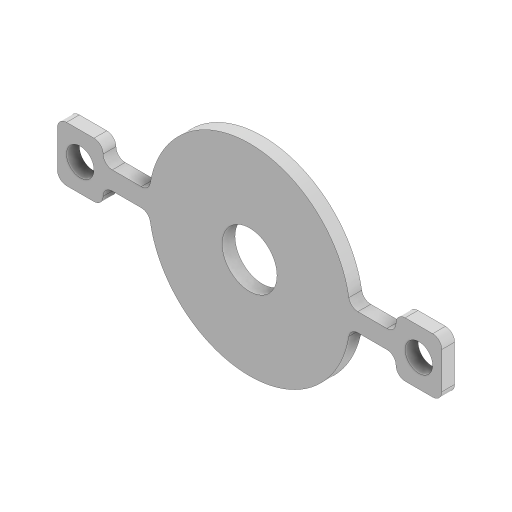
# Autodesk Inventor part: TAPA QUE DESPLAZA CON TORNILLOS
Saved by Autodesk Inventor 2024 (Build 280153000, 153)
## iProperties
Created: 2024-05-26
Part Number: TAPA QUE DESPLAZA CON TORNILLOS
Material: Generic
Document SubType Name: Modeling
Designer: Jhuliams
Density: 1 g/cm^3
Appearance: Default
Author: Jhuliams
Autodesk Inventor part; units mm, degrees
ref_plane "YZ Plane" through (0, 0, 0) normal (1, 0, 0) x (0, 1, 0)
ref_plane "XZ Plane" through (0, 0, 0) normal (0, 1, 0) x (-1, 0, 0)
ref_plane "XY Plane" through (0, 0, 0) normal (0, 0, 1) x (1, 0, 0)
sketch "Sketch1" plane through (0, 0, 0) normal (0, 0, 1) x (1, 0, 0)
  circle A0 centre (0, 0) radius 55
  line L0 (0, 0) -> (0, 20) construction
  line L1 (5, 15) -> (105, 15)
  line L2 (105, 15) -> (105, -15)
  line L3 (105, -15) -> (5, -15)
  line L4 (5, -15) -> (5, 15)
  line L5 (5, 15) -> (105, -15) construction
  line L6 (105, 15) -> (5, -15) construction
  line L7 (30, 5) -> (80, 5)
  line L8 (80, 5) -> (80, -5)
  line L9 (80, -5) -> (30, -5)
  line L10 (30, -5) -> (30, 5)
  line L11 (30, 5) -> (80, -5) construction
  line L12 (80, 5) -> (30, -5) construction
  line L13 (80, 5) -> (80, 15)
  line L14 (80, -5) -> (80, -15)
  line L15 (-5, 15) -> (-105, 15)
  line L16 (-105, 15) -> (-105, -15)
  line L17 (-105, -15) -> (-5, -15)
  line L18 (-5, -15) -> (-5, 15)
  line L19 (-5, 15) -> (-105, -15) construction
  line L20 (-105, 15) -> (-5, -15) construction
  line L21 (-30, 5) -> (-80, 5)
  line L22 (-80, 5) -> (-80, -5)
  line L23 (-80, -5) -> (-30, -5)
  line L24 (-30, -5) -> (-30, 5)
  line L25 (-30, 5) -> (-80, -5) construction
  line L26 (-80, 5) -> (-30, -5) construction
  line L27 (-80, 5) -> (-80, 15)
  line L28 (-80, -5) -> (-80, -15)
  point P0 (55, 0)
  point P1 (55, 0)
  point P2 (-55, 0)
  point P3 (-55, 0)
  point P4 (54.7723, 5)
  point P5 (54.7723, -5)
  point P6 (-54.7723, -5)
  point P7 (-54.7723, 5)
  dimension "d0" = 110
  dimension "d3" = 20
  dimension "d17" = 100
  dimension "d18" = 30
  dimension "d19" = 50
  dimension "d20" = 10
  constraints: 58 end point, 12 symmetric about line, 5 midpoint, 4 parallel, 4 perpendicular, 4 point on line, 2 horizontal, 1 coincident, 1 vertical, 3 other
  measures "d3" distance of L0.start L0.end
  measures "d17" distance of L2.end L3.end
  measures "d18" distance of L1.end L2.end
  measures "d19" distance of L8.end L9.end
  measures "d20" distance of L7.end L8.end
extrude "Extrusion1" add sketch "Sketch1" along normal blind 7 contours A0 L9 L10 L7 | A0 L7 L8 L9 | L7 L10 L9 A0 L3 L4 L1 | L1 L4 L3 A0 L17 L18 L15 | L13 L1 L2 L3 L14 L8 | L15 L18 L17 A0 L23 L24 L21 | L21 L24 L23 A0 | A0 L23 L22 L21 | L27 L22 L28 L17 L16 L15
sketch "Sketch2" plane through (0, 0, 7) normal (0, 0, 1) x (1, 0, 0)
  line L0 (0, 0) -> (-92.5, 0) construction
  circle A0 centre (-92.5, 0) radius 7.5
  line L1 (0, 0) -> (0, 20) construction
  circle A1 centre (92.5, 0) radius 7.5
  dimension "d6" = 92.5
  dimension "d7" = 15
  dimension "d8" = 20
  constraints: 4 end point, 2 centre point, 2 coincident, 2 symmetric about line, 1 horizontal, 1 vertical, 1 other
  measures "d6" distance of L0.start L0.end
  measures "d7" diameter of A0
  measures "d8" distance of L0.start L1.end
extrude "Extrusion2" cut sketch "Sketch2" against normal blind 7
fillet "Fillet1" radius 5 16 edges at (-80, 5, 3.5) (-80, 15, 3.5) (-54.7723, 5, 3.5) (-80, -5, 3.5) (-80, -15, 3.5) (-54.7723, -5, 3.5) (-105, -15, 3.5) (-105, 15, 3.5) (105, 15, 3.5) (105, -15, 3.5) (80, -15, 3.5) (80, 15, 3.5) (80, -5, 3.5) (80, 5, 3.5) (54.7723, 5, 3.5) (54.7723, -5, 3.5)
sketch "Sketch4" plane through (0, 0, 7) normal (0, 0, 1) x (1, 0, 0)
  circle A0 centre (0, 0) radius 15
  dimension "d14" = 30
  constraints: 1 centre point, 1 coincident
  measures "d14" diameter of A0
extrude "Extrusion3" cut sketch "Sketch4" against normal blind 10
body "Solid1"
